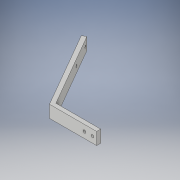
# Autodesk Inventor part: CollectionAngleBracket
Saved by Autodesk Inventor 2017 (Build 210142000, 142)
## iProperties
Created: 2018-06-09
Part Number: CollectionAngleBracket
Material: Generic
Document SubType Name: Modeling
Designer: User
Density: 1 g/cm^3
Appearance: Default
Author: User
Autodesk Inventor part; units mm, degrees
ref_plane "YZ Plane" through (0, 0, 0) normal (1, 0, 0) x (0, 1, 0)
ref_plane "XZ Plane" through (0, 0, 0) normal (0, 1, 0) x (-1, 0, 0)
ref_plane "XY Plane" through (0, 0, 0) normal (0, 0, 1) x (1, 0, 0)
sketch "Sketch1" plane through (0, 0, 0) normal (0, 1, 0) x (-1, 0, 0)
  line L0 (0, 0) -> (67.8242, -117.475)
  line L1 (0, 0) -> (135.6484, 0) construction
  line L2 (67.8242, -117.475) -> (62.325, -120.65)
  line L3 (62.325, -120.65) -> (-3.6662, -6.35)
  line L4 (-0.56, 0) -> (-73.5162, 0)
  line L5 (-73.5162, 0) -> (-73.5162, -6.35)
  line L6 (-3.6662, -6.35) -> (-73.5162, -6.35)
  line L7 (0, 0) -> (-0.56, 0)
  dimension "d0" = 60
  dimension "d2" = 6.35
  dimension "d3" = 6.35
  dimension "d4" = 0
  dimension "d5" = 114.3
  dimension "d6" = 69.85
  constraints: 16 end point, 3 horizontal, 3 perpendicular, 1 equal length
  measures "d0" angle of L0 L1
  measures "d2" distance between parallel lines of L3 L0
  measures "d3" distance of L4.end L5.end
  measures "d4" distance between parallel lines of L4 L1
  measures "d5" distance from line of L6 L2.end
  measures "d6" distance from line of L3.end L5
extrude "Extrusion1" add sketch "Sketch1" along normal blind 19.05
sketch "Sketch2" plane through (0, 0, 0) normal (0, 0, 1) x (1, 0, 0)
  line L0 (73.5162, 0) -> (0, 0) projected
  line L1 (73.5162, 0) -> (73.5162, 19.05) projected
  line L2 (0, 19.05) -> (73.5162, 19.05) projected
  line L3 (0, 0) -> (0, 19.05) projected
  point P0 (67.1662, 9.525)
  point P1 (54.4662, 9.525)
  dimension "d9" = 6.35
  dimension "d10" = 19.05
  dimension "d11" = 9.525
  dimension "d12" = 9.525
  measures "d9" distance from line of L1 point (67.166, 9.525)
  measures "d10" distance from line of L1 point (54.466, 9.525)
  measures "d11" distance from line of L0 point (67.166, 9.525)
  measures "d12" distance from line of L0 point (54.466, 9.525)
hole "Hole1" at (67.1662, 9.525, 0) at (54.4662, 9.525, 0) direction (0, 0, -1) diameter 4.445 end through all
sketch "Sketch3" plane through (0, 0, 0) normal (-0.8660254, 0, 0.5) x (0.5, 0, 0.8660254)
  line L0 (0, 0) -> (-135.6484, 0) projected
  line L1 (0, 0) -> (0, 19.05) projected
  line L2 (-135.6484, 19.05) -> (0, 19.05) projected
  line L3 (-135.6484, 0) -> (-135.6484, 19.05) projected
  point P0 (-129.2984, 9.525)
  point P1 (-91.1984, 9.525)
  dimension "d20" = 6.35
  dimension "d21" = 44.45
  dimension "d22" = 9.525
  dimension "d23" = 9.525
  measures "d20" distance from line of L3 point (-129.298, 9.525)
  measures "d21" distance from line of L3 point (-91.198, 9.525)
  measures "d22" distance from line of L2 point (-129.298, 9.525)
  measures "d23" distance from line of L2 point (-91.198, 9.525)
hole "Hole2" at (-64.6492, 9.525, -111.9757) at (-45.5992, 9.525, -78.9802) direction (0.8660254, 0, -0.5) diameter 4.064 end through all
equation "\"d12\" = d11"
body "Solid1"
